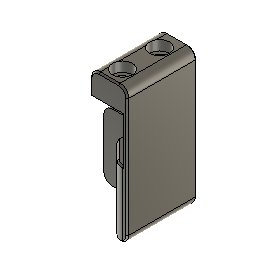
Encoder_Mount (Autodesk Fusion 360 design; units mm, degrees)
Autodesk Fusion 360 part; units mm, degrees
sketch "Sketch1" plane through (0, 0, 0) normal (0, 0, 1) x (1, 0, 0)
  line L0 (-6, 21) -> (-6, 6) construction
  circle A0 centre (-6, 6) radius 2.5
  circle A1 centre (-6, 21) radius 2.5
  circle A2 centre (-6, 6) radius 4
  circle A3 centre (-6, 21) radius 4
  dimension "d1" = 15
  dimension "d2" = 5
  dimension "d3" = 6
  dimension "d4" = 6
  dimension "d38" = 8
  constraint vertical L0
  constraint coincident L0.end A0.centre
  constraint coincident L0.start A1.centre
  constraint equal A0 A1
  constraint concentric A0 A2
  constraint concentric A1 A3
  constraint equal A2 A3
  measures "d1" distance of L0.start L0.end
  measures "d2" diameter of A1
  measures "d3" horizontal distance of origin L0.end
  measures "d4" vertical distance of origin L0.end
  measures "d38" diameter of A3
sketch "Sketch3" plane through (0, 0, 0) normal (1, 0, 0) x (0, 1, 0)
  line L0 (0, 10) -> (28, 10)
  line L1 (28, 10) -> (28, -18)
  line L2 (28, -18) -> (0, -18)
  line L3 (0, -18) -> (0, 10)
  line L4 (28, -18) -> (28, -45)
  line L5 (28, -45) -> (18, -45)
  line L6 (18, -45) -> (18, -18)
  dimension "d6" = 18
  dimension "d7" = 10
  dimension "d8" = 28
  dimension "d9" = 27
  dimension "d10" = 10
  constraint horizontal L0
  constraint vertical L1
  constraint horizontal L2
  constraint vertical L3
  constraint coincident L3 origin
  constraint perpendicular L2 L4
  constraint coincident L2 L6.end
  constraint perpendicular L5 L6
  constraint vertical L6
  measures "d6" distance of L2.end origin
  measures "d7" distance of L0.start origin
  measures "d8" distance of L0.start L0.end
  measures "d9" distance of L1.end L4.end
  measures "d10" distance of L4.end L5.end
sketch "Sketch4" plane through (0, 0, 0) normal (0, 1, 0) x (1, 0, 0)
  line L0 (0, 18) -> (0, -10)
  line L1 (0, 45) -> (0, 18)
  line L2 (-13, -10) -> (0, -10)
  line L3 (0, -10) -> (0, 18)
  line L4 (-13, 0) -> (-13, -10)
  line L5 (0, -10) -> (2, -10)
  line L6 (0, 45) -> (2, 45)
  line L7 (0, 0) -> (-13, 0)
  line L8 (0, 18) -> (-25.5, 18)
  line L9 (-25.5, 18) -> (-25.5, 45)
  line L10 (-25.5, 45) -> (0, 45)
  line L11 (-10.2, 18) -> (-10.2, 45)
  line L12 (-14, 22.5) -> (-14, 39.5) construction
  circle A0 centre (-14, 22.5) radius 1.3
  circle A1 centre (-14, 39.5) radius 1.3
  line L13 (2, -10) -> (2, 45)
  point P0 (0, 18)
  point P1 (-4, 45)
  dimension "d11" = 13
  dimension "d12" = 2
  dimension "d18" = 25.5
  dimension "d19" = 15.3
  dimension "d20" = 17
  dimension "d21" = 2.6
  dimension "d22" = 4.5
  dimension "d23" = 11.5
  dimension "d28" = 4
  constraint horizontal L2
  constraint vertical L3
  constraint vertical L4
  constraint coincident L0.end L2.end
  constraint coincident P0 L0.start
  constraint perpendicular L0 L5
  constraint coincident L1.start L6.start
  constraint perpendicular L1 L6
  constraint vertical L5.end L6.end
  constraint coincident L7.start origin
  constraint perpendicular L4 L7
  constraint perpendicular L0 L8
  constraint perpendicular L8 L9
  constraint horizontal L10
  constraint coincident L8 L11.start
  constraint coincident L10 L11.end
  constraint perpendicular L10 L11
  constraint perpendicular L8 L12
  constraint coincident L12.start A0.centre
  constraint coincident L12.end A1.centre
  constraint equal A0 A1
  constraint coincident L10 P1
  measures "d11" distance of L2.start L0.end
  measures "d12" distance of L1.start L6.end
  measures "d18" distance of L1.start L9.end
  measures "d19" distance of L9 L11
  measures "d20" distance of L12.start L12.end
  measures "d21" diameter of A0
  measures "d22" distance of L8 L12.start
  measures "d23" horizontal distance of L8.end L12.start
  measures "d28" distance of L1.start P1
extrude "Extrude1" add sketch "Sketch4" along normal up to surface (28 mm away) contours L0 L2 L3 L4 L7
extrude "Extrude2" add sketch "Sketch4" along normal up to surface (28 mm away) contours L0 L1 L3 L5 L6 L13 | L1 L8 L10 L11 | L8 L9 L10 L11 | A0 | A1
extrude "Extrude3" cut sketch "Sketch4" along normal up to surface (18 mm away) contours L8 L9 L10 L11 | A0 | A1
extrude "Extrude5" cut sketch "Sketch4" along normal blind 8 from surface at 18 contours A0 | A1
sketch "Sketch5" plane through (0, 0, -45) normal (0, 0, -1) x (1, 0, 0)
  line L0 (-10.2, -18) -> (-25.5, -18)
  line L1 (-25.5, -18) -> (-25.5, -28)
  line L2 (-25.5, -28) -> (2, -28)
  line L3 (2, 0) -> (-10.2, 0)
  line L4 (-10.2, 0) -> (-10.2, -18)
  line L5 (2, -24) -> (-10.2, -8)
  line L6 (2, -28) -> (2, 0)
  arc A0 (2, -24) -> (-10.2, -8) centre (-10.1602, -20.6209) ccw
  point P0 (-10.2, 0)
  point P1 (-4, 0)
  point P2 (0, -18)
  point P3 (0, -18)
  dimension "d27" = 4
  dimension "d45" = 10
  dimension "d46" = 5
  constraint vertical L2.end L5.start
  constraint vertical L5.end P0
  measures "d27" distance of L2.end L5.start
  measures "d45" vertical distance of L5.end P3
  measures "d46" distance of L5 A0
ref_plane "WorkPlane2" through (0, 0, 10) normal (0, 0, 1) x (1, 0, 0)
sketch "Sketch6" plane through (0, 0, 10) normal (0, 0, 1) x (1, 0, 0)
  line L0 (-2, 0) -> (2, 24)
  point P0 (0, 28)
  point P1 (0, 28)
  point P2 (2, 0)
  dimension "d30" = 4
  dimension "d31" = 4
  constraint vertical L0.end P2
  constraint horizontal L0.start P2
  measures "d30" vertical distance of L0.end P1
  measures "d31" horizontal distance of L0.start P2
ref_plane "WorkPlane1" through (0, 0, -18) normal (0, 0, 1) x (1, 0, 0)
extrude "Extrude4" cut sketch "Sketch1" along normal through all contours A0 | A1
extrude "Extrude6" cut sketch "Sketch1" along normal through all from surface at 6
chamfer "Chamfer2" distance 0.3 distance2 2 2 edges at (-15.212, 18, -22.0299) (-15.212, 18, -39.0299) measured on face at (-22.0247, 18, -33.9226) measured on face at (-22.0247, 18, -33.9226)
chamfer "Chamfer3" distance 8 distance2 8 1 edges at (-10.2, 0, -31.5) measured on face at (-2.7333, 0, -36)
fillet "Fillet3" chord length 5 5 edges at (2, 14, 10) (2, 14, -45) (-25.5, 23, -45) (-25.5, 23, -18) (-13, 14, 10)
fillet "Fillet3" chord length 4 1 edges at (-2.2, 0, -31.5)
chamfer "Chamfer4" distance 0.6 angle 45 4 faces at (-15.1548, 28, -36) (-3.6667, 0, 6.6667) (-1.0772, 0.1049, -26.9919) (-5.8872, 3.6872, -36)
